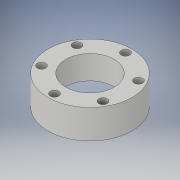
# Autodesk Inventor part: Adapter1
Saved by Autodesk Inventor 2019.3 (Build 233278000, 278)
## iProperties
Created: 2019-01-02
Part Number: Adapter1
Material: Generic
Document SubType Name: Modeling
Designer: eroldan
Density: 1 g/cm^3
Appearance: Default
Author: eroldan
Autodesk Inventor part; units mm, degrees
ref_plane "YZ Plane" through (0, 0, 0) normal (1, 0, 0) x (0, 1, 0)
ref_plane "XZ Plane" through (0, 0, 0) normal (0, 1, 0) x (-1, 0, 0)
ref_plane "XY Plane" through (0, 0, 0) normal (0, 0, 1) x (1, 0, 0)
sketch "Sketch3" plane through (0, 0, 0) normal (0, 0, 1) x (1, 0, 0)
  line L0 (26, 0) -> (21.75, 0.3)
  line L1 (26, 0) -> (26, 18)
  line L2 (21.75, 0.3) -> (21.75, 3.3)
  line L3 (21.75, 3.3) -> (15, 3.3)
  line L4 (15, 3.3) -> (15, 18)
  line L5 (15, 18) -> (26, 18)
  line L6 (0, -3.6) -> (0, 21.6) projected
  point P0 (0, 0)
  dimension "d5" = 26
  dimension "d6" = 21.75
  dimension "d7" = 0.3
  dimension "d8" = 18
  dimension "d9" = 15
  dimension "d10" = 3
  constraints: 12 end point, 3 vertical, 2 perpendicular, 1 horizontal alignment
  measures "d5" distance of L0.start point (0, 0)
  measures "d6" horizontal distance of L0.end point (0, 0)
  measures "d7" vertical distance of L0.start L0.end
  measures "d8" distance of L0.start L1.end
  measures "d9" horizontal distance of point (0, 0) L3.end
  measures "d10" vertical distance of L0.end L3.end
revolve "Revolution1" add sketch "Sketch3" angle 360 about axis through (0, -10, 0) along (0, 1, 0)
sketch "Sketch4" plane through (0, 18, 0) normal (0, 1, 0) x (1, 0, 0)
  point P0 (0, 0)
  point P1 (0, 22)
  point P2 (-19.0526, 11)
  point P3 (-19.0526, -11)
  point P4 (0, -22)
  point P5 (19.0526, -11)
  point P6 (19.0526, 11)
  dimension "d12" = 22
  dimension "d15" = 360
  constraints: 7 other
  measures "d12" distance of point (0, 0) point (0, 22)
hole "Hole1" at (0, 18, -22) at (-19.0526, 18, -11) at (-19.0526, 18, 11) at (0, 18, 22) at (19.0526, 18, 11) at (19.0526, 18, -11) direction (0, -1, 0) diameter 5.25 end through all both
body "Solid2"
